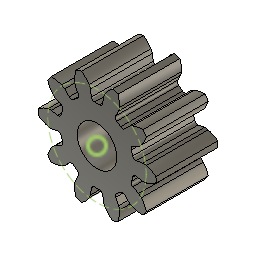
autopill_gear (Autodesk Fusion 360 design; units mm, degrees)
description: Spur Gear; Module: 1.270000; Number of Teeth: 10; Pressure Angle: 20.000000; Root Fillet Radius: 0.040000; Clearance: 0.000000; Gear Thickness: 0.800000; Hole Diameter: 0.510000;
Autodesk Fusion 360 part; units mm, degrees
sketch "Sketch1" plane through (0, 0, 0) normal (0, 1, 0) x (1, 0, 0) in component "Spur Gear (10 teeth)"
  arc A0 (4.4247, -1.7616) -> (4.6151, -1.1757) centre (0, 0) ccw
  arc A1 (5.0711, -0.8803) -> (4.6151, -1.1757) centre (5.0027, -1.2744) ccw
  line L0 (5.0711, -0.8803) -> (5.8986, -1.024)
  spline S0 degree 3 poles (5.8986, -1.024) (5.9495, -1.0286) (6.1022, -1.0345) (6.3611, -0.9743) knots 0 0 0 0 1 1 1 1
  spline S1 degree 3 poles (6.3611, -0.9743) (6.6663, -0.9023) (7.1002, -0.7379) (7.6128, -0.3728) knots 0 0 0 0 1 1 1 1
  arc A2 (7.6128, -0.3728) -> (7.6128, 0.3728) centre (0, 0) ccw
  spline S2 degree 3 poles (7.6128, 0.3728) (7.1002, 0.7379) (6.6663, 0.9023) (6.3611, 0.9743) knots 0 0 0 0 1 1 1 1
  spline S3 degree 3 poles (6.3611, 0.9743) (6.1022, 1.0345) (5.9495, 1.0286) (5.8986, 1.024) knots 0 0 0 0 1 1 1 1
  line L1 (5.8986, 1.024) -> (5.0711, 0.8803)
  arc A3 (4.6151, 1.1757) -> (5.0711, 0.8803) centre (5.0027, 1.2744) ccw
  arc A4 (4.6151, 1.1757) -> (4.4247, 1.7616) centre (0, 0) ccw
  arc A5 (4.6201, 2.2686) -> (4.4247, 1.7616) centre (4.7964, 1.9095) ccw
  line L2 (4.6201, 2.2686) -> (5.374, 2.6387)
  spline S4 degree 3 poles (5.374, 2.6387) (5.4179, 2.6649) (5.5448, 2.7499) (5.7189, 2.9507) knots 0 0 0 0 1 1 1 1
  spline S5 degree 3 poles (5.7189, 2.9507) (5.9235, 3.1884) (6.1779, 3.5764) (6.378, 4.1731) knots 0 0 0 0 1 1 1 1
  arc A6 (6.378, 4.1731) -> (5.9398, 4.7763) centre (0, 0) ccw
  spline S6 degree 3 poles (5.9398, 4.7763) (5.3104, 4.7704) (4.8628, 4.6484) (4.5736, 4.5272) knots 0 0 0 0 1 1 1 1
  spline S7 degree 3 poles (4.5736, 4.5272) (4.3287, 4.4237) (4.2087, 4.3292) (4.1702, 4.2955) knots 0 0 0 0 1 1 1 1
  line L3 (4.1702, 4.2955) -> (3.5852, 3.6929)
  arc A7 (3.0427, 3.6638) -> (3.5852, 3.6929) centre (3.2982, 3.9716) ccw
  arc A8 (3.0427, 3.6638) -> (2.5443, 4.0259) centre (0, 0) ccw
  arc A9 (2.4043, 4.5509) -> (2.5443, 4.0259) centre (2.758, 4.3641) ccw
  line L4 (2.4043, 4.5509) -> (2.7966, 5.2935)
  spline S8 degree 3 poles (2.7966, 5.2935) (2.8168, 5.3405) (2.8695, 5.4839) (2.8923, 5.7487) knots 0 0 0 0 1 1 1 1
  spline S9 degree 3 poles (2.8923, 5.7487) (2.9182, 6.0612) (2.8959, 6.5246) (2.707, 7.125) knots 0 0 0 0 1 1 1 1
  arc A10 (2.707, 7.125) -> (1.998, 7.3554) centre (0, 0) ccw
  spline S10 degree 3 poles (1.998, 7.3554) (1.4923, 6.9807) (1.2018, 6.6189) (1.0391, 6.3509) knots 0 0 0 0 1 1 1 1
  spline S11 degree 3 poles (1.0391, 6.3509) (0.9018, 6.1232) (0.8602, 5.9762) (0.8489, 5.9264) knots 0 0 0 0 1 1 1 1
  line L5 (0.8489, 5.9264) -> (0.7298, 5.095)
  arc A11 (0.308, 4.7525) -> (0.7298, 5.095) centre (0.3339, 5.1517) ccw
  arc A12 (0.308, 4.7525) -> (-0.308, 4.7525) centre (0, 0) ccw
  arc A13 (-0.7298, 5.095) -> (-0.308, 4.7525) centre (-0.3339, 5.1517) ccw
  line L6 (-0.7298, 5.095) -> (-0.8489, 5.9264)
  spline S12 degree 3 poles (-0.8489, 5.9264) (-0.8602, 5.9762) (-0.9018, 6.1232) (-1.0391, 6.3509) knots 0 0 0 0 1 1 1 1
  spline S13 degree 3 poles (-1.0391, 6.3509) (-1.2018, 6.6189) (-1.4923, 6.9807) (-1.998, 7.3554) knots 0 0 0 0 1 1 1 1
  arc A14 (-1.998, 7.3554) -> (-2.707, 7.125) centre (0, 0) ccw
  spline S14 degree 3 poles (-2.707, 7.125) (-2.8959, 6.5246) (-2.9182, 6.0612) (-2.8923, 5.7487) knots 0 0 0 0 1 1 1 1
  spline S15 degree 3 poles (-2.8923, 5.7487) (-2.8695, 5.4839) (-2.8168, 5.3405) (-2.7966, 5.2935) knots 0 0 0 0 1 1 1 1
  line L7 (-2.7966, 5.2935) -> (-2.4043, 4.5509)
  arc A15 (-2.5443, 4.0259) -> (-2.4043, 4.5509) centre (-2.758, 4.3641) ccw
  arc A16 (-2.5443, 4.0259) -> (-3.0427, 3.6638) centre (0, 0) ccw
  arc A17 (-3.5852, 3.6929) -> (-3.0427, 3.6638) centre (-3.2982, 3.9716) ccw
  line L8 (-3.5852, 3.6929) -> (-4.1702, 4.2955)
  spline S16 degree 3 poles (-4.1702, 4.2955) (-4.2087, 4.3292) (-4.3287, 4.4237) (-4.5736, 4.5272) knots 0 0 0 0 1 1 1 1
  spline S17 degree 3 poles (-4.5736, 4.5272) (-4.8628, 4.6484) (-5.3104, 4.7704) (-5.9398, 4.7763) knots 0 0 0 0 1 1 1 1
  arc A18 (-5.9398, 4.7763) -> (-6.378, 4.1731) centre (0, 0) ccw
  spline S18 degree 3 poles (-6.378, 4.1731) (-6.1779, 3.5764) (-5.9235, 3.1884) (-5.7189, 2.9507) knots 0 0 0 0 1 1 1 1
  spline S19 degree 3 poles (-5.7189, 2.9507) (-5.5448, 2.7499) (-5.4179, 2.6649) (-5.374, 2.6387) knots 0 0 0 0 1 1 1 1
  line L9 (-5.374, 2.6387) -> (-4.6201, 2.2686)
  arc A19 (-4.4247, 1.7616) -> (-4.6201, 2.2686) centre (-4.7964, 1.9095) ccw
  arc A20 (-4.4247, 1.7616) -> (-4.6151, 1.1757) centre (0, 0) ccw
  arc A21 (-5.0711, 0.8803) -> (-4.6151, 1.1757) centre (-5.0027, 1.2744) ccw
  line L10 (-5.0711, 0.8803) -> (-5.8986, 1.024)
  spline S20 degree 3 poles (-5.8986, 1.024) (-5.9495, 1.0286) (-6.1022, 1.0345) (-6.3611, 0.9743) knots 0 0 0 0 1 1 1 1
  spline S21 degree 3 poles (-6.3611, 0.9743) (-6.6663, 0.9023) (-7.1002, 0.7379) (-7.6128, 0.3728) knots 0 0 0 0 1 1 1 1
  arc A22 (-7.6128, 0.3728) -> (-7.6128, -0.3728) centre (0, 0) ccw
  spline S22 degree 3 poles (-7.6128, -0.3728) (-7.1002, -0.7379) (-6.6663, -0.9023) (-6.3611, -0.9743) knots 0 0 0 0 1 1 1 1
  spline S23 degree 3 poles (-6.3611, -0.9743) (-6.1022, -1.0345) (-5.9495, -1.0286) (-5.8986, -1.024) knots 0 0 0 0 1 1 1 1
  line L11 (-5.8986, -1.024) -> (-5.0711, -0.8803)
  arc A23 (-4.6151, -1.1757) -> (-5.0711, -0.8803) centre (-5.0027, -1.2744) ccw
  arc A24 (-4.6151, -1.1757) -> (-4.4247, -1.7616) centre (0, 0) ccw
  arc A25 (-4.6201, -2.2686) -> (-4.4247, -1.7616) centre (-4.7964, -1.9095) ccw
  line L12 (-4.6201, -2.2686) -> (-5.374, -2.6387)
  spline S24 degree 3 poles (-5.374, -2.6387) (-5.4179, -2.6649) (-5.5448, -2.7499) (-5.7189, -2.9507) knots 0 0 0 0 1 1 1 1
  spline S25 degree 3 poles (-5.7189, -2.9507) (-5.9235, -3.1884) (-6.1779, -3.5764) (-6.378, -4.1731) knots 0 0 0 0 1 1 1 1
  arc A26 (-6.378, -4.1731) -> (-5.9398, -4.7763) centre (0, 0) ccw
  spline S26 degree 3 poles (-5.9398, -4.7763) (-5.3104, -4.7704) (-4.8628, -4.6484) (-4.5736, -4.5272) knots 0 0 0 0 1 1 1 1
  spline S27 degree 3 poles (-4.5736, -4.5272) (-4.3287, -4.4237) (-4.2087, -4.3292) (-4.1702, -4.2955) knots 0 0 0 0 1 1 1 1
  line L13 (-4.1702, -4.2955) -> (-3.5852, -3.6929)
  arc A27 (-3.0427, -3.6638) -> (-3.5852, -3.6929) centre (-3.2982, -3.9716) ccw
  arc A28 (-3.0427, -3.6638) -> (-2.5443, -4.0259) centre (0, 0) ccw
  arc A29 (-2.4043, -4.5509) -> (-2.5443, -4.0259) centre (-2.758, -4.3641) ccw
  line L14 (-2.4043, -4.5509) -> (-2.7966, -5.2935)
  spline S28 degree 3 poles (-2.7966, -5.2935) (-2.8168, -5.3405) (-2.8695, -5.4839) (-2.8923, -5.7487) knots 0 0 0 0 1 1 1 1
  spline S29 degree 3 poles (-2.8923, -5.7487) (-2.9182, -6.0612) (-2.8959, -6.5246) (-2.707, -7.125) knots 0 0 0 0 1 1 1 1
  arc A30 (-2.707, -7.125) -> (-1.998, -7.3554) centre (0, 0) ccw
  spline S30 degree 3 poles (-1.998, -7.3554) (-1.4923, -6.9807) (-1.2018, -6.6189) (-1.0391, -6.3509) knots 0 0 0 0 1 1 1 1
  spline S31 degree 3 poles (-1.0391, -6.3509) (-0.9018, -6.1232) (-0.8602, -5.9762) (-0.8489, -5.9264) knots 0 0 0 0 1 1 1 1
  line L15 (-0.8489, -5.9264) -> (-0.7298, -5.095)
  arc A31 (-0.308, -4.7525) -> (-0.7298, -5.095) centre (-0.3339, -5.1517) ccw
  arc A32 (-0.308, -4.7525) -> (0.308, -4.7525) centre (0, 0) ccw
  arc A33 (0.7298, -5.095) -> (0.308, -4.7525) centre (0.3339, -5.1517) ccw
  line L16 (0.7298, -5.095) -> (0.8489, -5.9264)
  spline S32 degree 3 poles (0.8489, -5.9264) (0.8602, -5.9762) (0.9018, -6.1232) (1.0391, -6.3509) knots 0 0 0 0 1 1 1 1
  spline S33 degree 3 poles (1.0391, -6.3509) (1.2018, -6.6189) (1.4923, -6.9807) (1.998, -7.3554) knots 0 0 0 0 1 1 1 1
  arc A34 (1.998, -7.3554) -> (2.707, -7.125) centre (0, 0) ccw
  spline S34 degree 3 poles (2.707, -7.125) (2.8959, -6.5246) (2.9182, -6.0612) (2.8923, -5.7487) knots 0 0 0 0 1 1 1 1
  spline S35 degree 3 poles (2.8923, -5.7487) (2.8695, -5.4839) (2.8168, -5.3405) (2.7966, -5.2935) knots 0 0 0 0 1 1 1 1
  line L17 (2.7966, -5.2935) -> (2.4043, -4.5509)
  arc A35 (2.5443, -4.0259) -> (2.4043, -4.5509) centre (2.758, -4.3641) ccw
  arc A36 (2.5443, -4.0259) -> (3.0427, -3.6638) centre (0, 0) ccw
  arc A37 (3.5852, -3.6929) -> (3.0427, -3.6638) centre (3.2982, -3.9716) ccw
  line L18 (3.5852, -3.6929) -> (4.1702, -4.2955)
  spline S36 degree 3 poles (4.1702, -4.2955) (4.2087, -4.3292) (4.3287, -4.4237) (4.5736, -4.5272) knots 0 0 0 0 1 1 1 1
  spline S37 degree 3 poles (4.5736, -4.5272) (4.8628, -4.6484) (5.3104, -4.7704) (5.9398, -4.7763) knots 0 0 0 0 1 1 1 1
  arc A38 (5.9398, -4.7763) -> (6.378, -4.1731) centre (0, 0) ccw
  spline S38 degree 3 poles (6.378, -4.1731) (6.1779, -3.5764) (5.9235, -3.1884) (5.7189, -2.9507) knots 0 0 0 0 1 1 1 1
  spline S39 degree 3 poles (5.7189, -2.9507) (5.5448, -2.7499) (5.4179, -2.6649) (5.374, -2.6387) knots 0 0 0 0 1 1 1 1
  line L19 (5.374, -2.6387) -> (4.6201, -2.2686)
  arc A39 (4.4247, -1.7616) -> (4.6201, -2.2686) centre (4.7964, -1.9095) ccw
  circle A40 centre (0, 0) radius 2.55
extrude "Extrude1" add sketch "Sketch1" along normal blind 8 in component "Spur Gear (10 teeth)"
sketch "Sketch2" plane through (0, 0, 0) normal (0, 1, 0) x (1, 0, 0) in component "Spur Gear (10 teeth)"
  circle A0 centre (0, 0) radius 6.35 construction
component "Spur Gear (10 teeth)" placed x (1, 0, 0) y (0, 1, 0) z (0, 0, 1) at (0, 0, 0)
